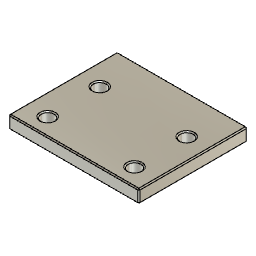
X Ballnut Spacer (Autodesk Fusion 360 design; units mm, degrees)
Autodesk Fusion 360 part; units mm, degrees
sketch "Sketch1" plane through (0, 0, 0) normal (0, 0, 1) x (1, 0, 0)
  line L0 (30, 25) -> (-30, 25)
  line L1 (-30, 25) -> (-30, -25)
  line L2 (-30, -25) -> (30, -25)
  line L3 (30, -25) -> (30, 25)
  line L4 (30, 25) -> (-30, -25) construction
  line L5 (-30, 25) -> (30, -25) construction
  line L6 (-20, 7) -> (20, 7) construction
  line L7 (20, 7) -> (20, -17) construction
  line L8 (20, -17) -> (-20, -17) construction
  line L9 (-20, -17) -> (-20, 7) construction
  circle A0 centre (-20, -17) radius 3
  circle A1 centre (20, -17) radius 3
  circle A2 centre (-20, 7) radius 3
  circle A3 centre (20, 7) radius 3
  dimension "d1" = 60
  dimension "d2" = 50
  dimension "d3" = 40
  dimension "d4" = 24
  dimension "d5" = 10
  dimension "d6" = 8
  dimension "d7" = 6
  dimension "d8" = 6
  dimension "d9" = 6
  dimension "d10" = 6
  constraint perpendicular L0 L1
  constraint parallel L0 L2
  constraint parallel L1 L3
  constraint horizontal L0
  constraint coincident L4 origin
  constraint coincident L5 origin
  constraint horizontal L6
  constraint vertical L7
  constraint horizontal L8
  constraint vertical L9
  constraint coincident L8.end L9.start
  constraint coincident L7.end L8.start
  constraint coincident L6.start L9.end
  constraint coincident L6.end L7.start
  measures "d1" distance of L1.end L2.end
  measures "d2" distance of L0.end L1.end
  measures "d3" distance of L6.start L6.end
  measures "d4" distance of L6.start L8.end
  measures "d5" distance of L3 L7
  measures "d6" distance of L2 L8
  measures "d7" diameter of A0
  measures "d8" diameter of A1
  measures "d9" diameter of A2
  measures "d10" diameter of A3
extrude "Extrude1" add sketch "Sketch1" along normal blind 6
chamfer "Chamfer1" distance 0.5 angle 45 20 edges at (-30, 0, 6) (-30, 25, 3) (0, 25, 6) (-30, -25, 3) (0, -25, 6) (0, -25, 0) (30, 25, 3) (0, 25, 0) (30, 0, 6) (30, 0, 0) (30, -25, 3) (-30, 0, 0) (-22.797, 8.0848, 6) (-22.797, 8.0848, 0) (-22.797, -15.9152, 6) (-22.797, -15.9152, 0) (17.203, -15.9152, 6) (17.203, -15.9152, 0) (17.203, 8.0848, 6) (17.203, 8.0848, 0)
equation "d5 = d1 / 2 - d3 / 2"
equation "d6 = 20 mm - d4 / 2"
named bodies: "Spacer plate"
